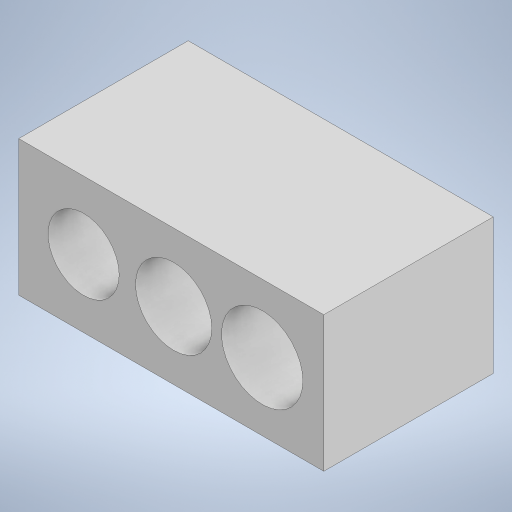
# Autodesk Inventor part: M5 size test for tapping
Saved by Autodesk Inventor 2023 (Build 270158000, 158)
## iProperties
Created: 2024-06-27
Part Number: M5 size test for tapping
Material: Generic
Document SubType Name: Modeling
Designer: Akramilab
Density: 1 g/cm^3
Appearance: Default
Author: Akramilab
Autodesk Inventor part; units mm, degrees
ref_plane "YZ Plane" through (0, 0, 0) normal (1, 0, 0) x (0, 1, 0)
ref_plane "XZ Plane" through (0, 0, 0) normal (0, 1, 0) x (-1, 0, 0)
ref_plane "XY Plane" through (0, 0, 0) normal (0, 0, 1) x (1, 0, 0)
sketch "Sketch6" plane through (0, 0, 0) normal (0, 0, 1) x (1, 0, 0)
  line L0 (0, 0) -> (18, 0)
  line L1 (18, 0) -> (18, -8)
  line L2 (18, -8) -> (0, -8)
  line L3 (0, -8) -> (0, 0)
  circle A0 centre (3.8277, -4) radius 2.1
  circle A1 centre (9.1415, -4) radius 2.25
  circle A2 centre (14.3653, -4) radius 2.4
  dimension "d11" = 18
  dimension "d12" = 8
  dimension "d13" = 4.2
  dimension "d14" = 4.5
  dimension "d15" = 4.8
  constraints: 8 end point, 3 centre point, 2 parallel, 1 horizontal, 1 perpendicular
  measures "d11" distance of L1.end L2.end
  measures "d12" distance of L0.end L1.end
  measures "d13" diameter of A0
  measures "d14" diameter of A1
  measures "d15" diameter of A2
extrude "Extrusion4" add sketch "Sketch6" along normal blind 10
body "Solid3"
